Autodesk Inventor part; units mm, degrees
(part 3 of 3)
sketch "Эскиз6" plane through (0, 2, 0) normal (0, 1, 0) x (1, 0, 0)
  circle A0 centre (0, -40) radius 1.6 construction
  circle A1 centre (-46, 0) radius 1.6 construction
  circle A2 centre (46, 0) radius 1.6 construction
  line L0 (-6.25948, 46.133514) -> (-19.274559, 46.133514) construction
  arc A3 (-19.274559, 46.133514) -> (-21.669819, 47.125663) centre (-21.92031, 43.133514) ccw construction
  line L1 (-21.669819, 47.125663) -> (-42.426407, 67.882251) construction
  line L2 (-42.426407, 67.882251) -> (-34.294679, 76.013979) construction
  arc A4 (-34.294679, 76.013979) -> (-34.294679, 83.085047) centre (-37.830213, 79.549513) ccw construction
  line L3 (-34.294679, 83.085047) -> (-38.389169, 87.179537) construction
  arc A5 (-37.745267, 90.439454) -> (-38.389169, 87.179537) centre (-36.974956, 88.593751) ccw construction
  arc A6 (-25.810185, 94.54012) -> (-37.745267, 90.439454) centre (0, 0) ccw construction
  arc A7 (-25.810185, 94.54012) -> (-20.747604, 95.778583) centre (-24, 98.107084) ccw construction
  arc A8 (20.747604, 95.778583) -> (-20.747604, 95.778583) centre (0, 0) ccw construction
  arc A9 (20.747604, 95.778583) -> (25.810185, 94.54012) centre (24, 98.107084) ccw construction
  arc A10 (37.745267, 90.439454) -> (25.810185, 94.54012) centre (0, 0) ccw construction
  arc A11 (38.389169, 87.179537) -> (37.745267, 90.439454) centre (36.974956, 88.593751) ccw construction
  line L4 (38.389169, 87.179537) -> (34.294679, 83.085047) construction
  arc A12 (34.294679, 83.085047) -> (34.294679, 76.013979) centre (37.830213, 79.549513) ccw construction
  line L5 (34.294679, 76.013979) -> (42.426407, 67.882251) construction
  line L6 (42.426407, 67.882251) -> (21.669819, 47.125663) construction
  arc A13 (21.669819, 47.125663) -> (19.274559, 46.133514) centre (21.92031, 43.133514) ccw construction
  line L7 (19.274559, 46.133514) -> (6.25948, 46.133514) construction
  arc A14 (3.576846, 47.790579) -> (6.25948, 46.133514) centre (6.25948, 49.133514) ccw construction
  arc A15 (3.576846, 47.790579) -> (-3.576846, 47.790579) centre (0, 46) ccw construction
  arc A16 (-6.25948, 46.133514) -> (-3.576846, 47.790579) centre (-6.25948, 49.133514) ccw construction
  arc A17 (48.648149, 93.050296) -> (-48.648149, 93.050296) centre (0, 0) ccw construction
  arc A18 (-48.648149, 93.050296) -> (-49.379523, 88.270396) centre (-47.258202, 90.391716) ccw construction
  line L8 (-49.379523, 88.270396) -> (-46.315494, 85.206367) construction
  arc A19 (-46.315494, 73.892659) -> (-46.315494, 85.206367) centre (-51.972348, 79.549513) ccw construction
  line L9 (-46.315494, 73.892659) -> (-73.892659, 46.315494) construction
  arc A20 (-85.206367, 46.315494) -> (-73.892659, 46.315494) centre (-79.549513, 51.972348) ccw construction
  line L10 (-85.206367, 46.315494) -> (-88.270396, 49.379523) construction
  arc A21 (-88.270396, 49.379523) -> (-93.050296, 48.648149) centre (-90.391716, 47.258202) ccw
  arc A22 (-93.050296, 48.648149) -> (-93.050296, -48.648149) centre (0, 0) ccw construction
  arc A23 (-93.050296, -48.648149) -> (-88.270396, -49.379523) centre (-90.391716, -47.258202) ccw
  line L11 (-88.270396, -49.379523) -> (-85.206367, -46.315494) construction
  arc A24 (-73.892659, -46.315494) -> (-85.206367, -46.315494) centre (-79.549513, -51.972348) ccw construction
  line L12 (-73.892659, -46.315494) -> (-46.315494, -73.892659) construction
  arc A25 (-46.315494, -85.206367) -> (-46.315494, -73.892659) centre (-51.972348, -79.549513) ccw construction
  line L13 (-46.315494, -85.206367) -> (-49.379523, -88.270396) construction
  arc A26 (-49.379523, -88.270396) -> (-48.648149, -93.050296) centre (-47.258202, -90.391716) ccw construction
  arc A27 (-48.648149, -93.050296) -> (-45.41996, -94.667984) centre (0, 0) ccw construction
  arc A28 (-45.41996, -94.667984) -> (-43.035533, -94.165467) centre (-44.554817, -92.864785) ccw construction
  line L14 (-43.035533, -94.165467) -> (-18.380184, -65.366371) construction
  arc A29 (-17.477038, -64.764325) -> (-18.380184, -65.366371) centre (-16.8609, -66.667053) ccw construction
  line L15 (-17.477038, -64.764325) -> (-0.616138, -59.304458) construction
  arc A30 (0.616138, -59.304458) -> (-0.616138, -59.304458) centre (0, -61.207186) ccw construction
  line L16 (0.616138, -59.304458) -> (17.477038, -64.764325) construction
  arc A31 (18.380184, -65.366371) -> (17.477038, -64.764325) centre (16.8609, -66.667053) ccw construction
  line L17 (18.380184, -65.366371) -> (43.035533, -94.165467) construction
  arc A32 (43.035533, -94.165467) -> (45.41996, -94.667984) centre (44.554817, -92.864785) ccw construction
  arc A33 (45.41996, -94.667984) -> (48.648149, -93.050296) centre (0, 0) ccw construction
  arc A34 (48.648149, -93.050296) -> (49.379523, -88.270396) centre (47.258202, -90.391716) ccw construction
  line L18 (49.379523, -88.270396) -> (46.315494, -85.206367) construction
  arc A35 (46.315494, -73.892659) -> (46.315494, -85.206367) centre (51.972348, -79.549513) ccw construction
  line L19 (46.315494, -73.892659) -> (73.892659, -46.315494) construction
  arc A36 (85.206367, -46.315494) -> (73.892659, -46.315494) centre (79.549513, -51.972348) ccw construction
  line L20 (85.206367, -46.315494) -> (88.270396, -49.379523) construction
  arc A37 (88.270396, -49.379523) -> (93.050296, -48.648149) centre (90.391716, -47.258202) ccw construction
  arc A38 (93.050296, -48.648149) -> (93.050296, 48.648149) centre (0, 0) ccw construction
  arc A39 (93.050296, 48.648149) -> (88.270396, 49.379523) centre (90.391716, 47.258202) ccw construction
  line L21 (88.270396, 49.379523) -> (85.206367, 46.315494) construction
  arc A40 (73.892659, 46.315494) -> (85.206367, 46.315494) centre (79.549513, 51.972348) ccw construction
  line L22 (73.892659, 46.315494) -> (46.315494, 73.892659) construction
  arc A41 (46.315494, 85.206367) -> (46.315494, 73.892659) centre (51.972348, 79.549513) ccw construction
  line L23 (46.315494, 85.206367) -> (49.379523, 88.270396) construction
  arc A42 (49.379523, 88.270396) -> (48.648149, 93.050296) centre (47.258202, 90.391716) ccw construction
  circle A43 centre (-24, 98.107084) radius 1.6 construction
  arc A44 (47.790579, -3.576846) -> (46.133514, -6.25948) centre (49.133514, -6.25948) ccw construction
  arc A45 (47.790579, -3.576846) -> (47.790579, 3.576846) centre (46, 0) ccw construction
  arc A46 (46.133514, 6.25948) -> (47.790579, 3.576846) centre (49.133514, 6.25948) ccw construction
  line L24 (46.133514, 6.25948) -> (46.133514, 19.274559) construction
  arc A47 (46.133514, 19.274559) -> (47.125663, 21.669819) centre (43.133514, 21.92031) ccw construction
  line L25 (47.125663, 21.669819) -> (67.882251, 42.426407) construction
  line L26 (67.882251, 42.426407) -> (76.013979, 34.294679) construction
  arc A48 (76.013979, 34.294679) -> (83.085047, 34.294679) centre (79.549513, 37.830213) ccw construction
  line L27 (83.085047, 34.294679) -> (87.179537, 38.389169) construction
  arc A49 (90.439454, 37.745267) -> (87.179537, 38.389169) centre (88.593751, 36.974956) ccw construction
  arc A50 (97.965347, 2.605931) -> (90.439454, 37.745267) centre (0, 0) ccw construction
  arc A51 (97.965347, 2.605931) -> (97.965347, -2.605931) centre (101, 0) ccw construction
  arc A52 (90.439454, -37.745267) -> (97.965347, -2.605931) centre (0, 0) ccw construction
  arc A53 (87.179537, -38.389169) -> (90.439454, -37.745267) centre (88.593751, -36.974956) ccw construction
  line L28 (87.179537, -38.389169) -> (83.085047, -34.294679) construction
  arc A54 (83.085047, -34.294679) -> (76.013979, -34.294679) centre (79.549513, -37.830213) ccw construction
  line L29 (76.013979, -34.294679) -> (67.882251, -42.426407) construction
  line L30 (67.882251, -42.426407) -> (47.125663, -21.669819) construction
  arc A55 (47.125663, -21.669819) -> (46.133514, -19.274559) centre (43.133514, -21.92031) ccw construction
  line L31 (46.133514, -19.274559) -> (46.133514, -6.25948) construction
  circle A56 centre (101, 0) radius 1.6 construction
  circle A57 centre (-101, 0) radius 1.6 construction
  arc A58 (-47.790579, 3.576846) -> (-46.133514, 6.25948) centre (-49.133514, 6.25948) ccw construction
  arc A59 (-47.790579, 3.576846) -> (-47.790579, -3.576846) centre (-46, 0) ccw construction
  arc A60 (-46.133514, -6.25948) -> (-47.790579, -3.576846) centre (-49.133514, -6.25948) ccw construction
  line L32 (-46.133514, -6.25948) -> (-46.133514, -19.274559) construction
  arc A61 (-46.133514, -19.274559) -> (-47.125663, -21.669819) centre (-43.133514, -21.92031) ccw construction
  line L33 (-47.125663, -21.669819) -> (-67.882251, -42.426407) construction
  line L34 (-67.882251, -42.426407) -> (-76.013979, -34.294679) construction
  arc A62 (-76.013979, -34.294679) -> (-83.085047, -34.294679) centre (-79.549513, -37.830213) ccw construction
  line L35 (-83.085047, -34.294679) -> (-87.179537, -38.389169) construction
  arc A63 (-90.439454, -37.745267) -> (-87.179537, -38.389169) centre (-88.593751, -36.974956) ccw construction
  arc A64 (-97.965347, -2.605931) -> (-90.439454, -37.745267) centre (0, 0) ccw construction
  arc A65 (-97.965347, -2.605931) -> (-97.965347, 2.605931) centre (-101, 0) ccw construction
  arc A66 (-90.439454, 37.745267) -> (-97.965347, 2.605931) centre (0, 0) ccw construction
  arc A67 (-87.179537, 38.389169) -> (-90.439454, 37.745267) centre (-88.593751, 36.974956) ccw construction
  line L36 (-87.179537, 38.389169) -> (-83.085047, 34.294679) construction
  arc A68 (-83.085047, 34.294679) -> (-76.013979, 34.294679) centre (-79.549513, 37.830213) ccw construction
  line L37 (-76.013979, 34.294679) -> (-67.882251, 42.426407) construction
  line L38 (-67.882251, 42.426407) -> (-47.125663, 21.669819) construction
  arc A69 (-47.125663, 21.669819) -> (-46.133514, 19.274559) centre (-43.133514, 21.92031) ccw construction
  line L39 (-46.133514, 19.274559) -> (-46.133514, 6.25948) construction
  circle A70 centre (45.111051, -90.365885) radius 1.6 construction
  circle A71 centre (45.111051, 90.365885) radius 1.6 construction
  circle A72 centre (90.365885, 45.111051) radius 1.6 construction
  circle A73 centre (-45.111051, -90.365885) radius 1.6 construction
  circle A74 centre (90.365885, -45.111051) radius 1.6 construction
  circle A75 centre (-45.111051, 90.365885) radius 1.6 construction
  circle A76 centre (-90.365885, 45.111051) radius 1.6 construction
  circle A77 centre (-90.365885, -45.111051) radius 1.6 construction
  line L40 (63.63961, 46.669048) -> (43.84062, 26.870058) construction
  arc A78 (41.012193, 26.870058) -> (43.84062, 26.870058) centre (42.426407, 28.284271) ccw construction
  line L41 (41.012193, 26.870058) -> (26.870058, 41.012193) construction
  arc A79 (26.870058, 43.84062) -> (26.870058, 41.012193) centre (28.284271, 42.426407) ccw construction
  line L42 (26.870058, 43.84062) -> (46.669048, 63.63961) construction
  line L43 (46.669048, 63.63961) -> (63.63961, 46.669048) construction
  line L44 (-46.669048, 63.63961) -> (-26.870058, 43.84062) construction
  arc A80 (-26.870058, 41.012193) -> (-26.870058, 43.84062) centre (-28.284271, 42.426407) ccw construction
  line L45 (-26.870058, 41.012193) -> (-41.012193, 26.870058) construction
  arc A81 (-43.84062, 26.870058) -> (-41.012193, 26.870058) centre (-42.426407, 28.284271) ccw construction
  line L46 (-43.84062, 26.870058) -> (-63.63961, 46.669048) construction
  line L47 (-63.63961, 46.669048) -> (-46.669048, 63.63961) construction
  line L48 (-63.63961, -46.669048) -> (-43.84062, -26.870058) construction
  arc A82 (-41.012193, -26.870058) -> (-43.84062, -26.870058) centre (-42.426407, -28.284271) ccw construction
  line L49 (-41.012193, -26.870058) -> (-26.870058, -41.012193) construction
  arc A83 (-26.870058, -43.84062) -> (-26.870058, -41.012193) centre (-28.284271, -42.426407) ccw construction
  line L50 (-26.870058, -43.84062) -> (-46.669048, -63.63961) construction
  line L51 (-46.669048, -63.63961) -> (-63.63961, -46.669048) construction
  line L52 (-42.426407, -67.882251) -> (-21.669819, -47.125663) construction
  arc A84 (-21.669819, -47.125663) -> (-19.274559, -46.133514) centre (-21.92031, -43.133514) ccw construction
  line L53 (-19.274559, -46.133514) -> (19.274559, -46.133514) construction
  arc A85 (19.274559, -46.133514) -> (21.669819, -47.125663) centre (21.92031, -43.133514) ccw construction
  line L54 (21.669819, -47.125663) -> (42.426407, -67.882251) construction
  line L55 (42.426407, -67.882251) -> (37.124381, -73.184277) construction
  arc A86 (34.190883, -73.070746) -> (37.124381, -73.184277) centre (35.710168, -71.770063) ccw construction
  line L56 (34.190883, -73.070746) -> (25.418693, -62.824241) construction
  arc A87 (24.841986, -61.889251) -> (25.418693, -62.824241) centre (28.115423, -60.51553) ccw construction
  line L57 (24.841986, -61.889251) -> (23.83128, -59.480842) construction
  arc A88 (23.83128, -59.480842) -> (21.004883, -57.332824) centre (20.557843, -60.854564) ccw construction
  line L58 (21.004883, -57.332824) -> (15.158499, -56.590699) construction
  arc A89 (14.511894, -56.446301) -> (15.158499, -56.590699) centre (15.605539, -53.068959) ccw construction
  line L59 (14.511894, -56.446301) -> (0.616138, -51.946601) construction
  arc A90 (0.616138, -51.946601) -> (-0.616138, -51.946601) centre (0, -53.849329) ccw construction
  line L60 (-0.616138, -51.946601) -> (-14.511894, -56.446301) construction
  arc A91 (-15.158499, -56.590699) -> (-14.511894, -56.446301) centre (-15.605539, -53.068959) ccw construction
  line L61 (-15.158499, -56.590699) -> (-21.004883, -57.332824) construction
  arc A92 (-21.004883, -57.332824) -> (-23.83128, -59.480842) centre (-20.557843, -60.854564) ccw construction
  line L62 (-23.83128, -59.480842) -> (-24.841986, -61.889251) construction
  arc A93 (-25.418693, -62.824241) -> (-24.841986, -61.889251) centre (-28.115423, -60.51553) ccw construction
  line L63 (-25.418693, -62.824241) -> (-34.190883, -73.070746) construction
  arc A94 (-37.124381, -73.184277) -> (-34.190883, -73.070746) centre (-35.710168, -71.770063) ccw construction
  line L64 (-37.124381, -73.184277) -> (-42.426407, -67.882251) construction
  circle A95 centre (43.133514, 21.92031) radius 1.6 construction
  circle A96 centre (21.92031, -43.133514) radius 1.6 construction
  circle A97 centre (-21.92031, -43.133514) radius 1.6 construction
  circle A98 centre (-43.133514, -21.92031) radius 1.6 construction
  circle A99 centre (-43.133514, 21.92031) radius 1.6 construction
  circle A100 centre (-21.92031, 43.133514) radius 1.6 construction
  circle A101 centre (43.133514, -21.92031) radius 1.6 construction
  circle A102 centre (21.92031, 43.133514) radius 1.6 construction
  circle A103 centre (-37.830213, 79.549513) radius 1.6 construction
  circle A104 centre (-79.549513, 37.830213) radius 1.6 construction
  circle A105 centre (-79.549513, -37.830213) radius 1.6 construction
  circle A106 centre (79.549513, -37.830213) radius 1.6 construction
  circle A107 centre (37.830213, 79.549513) radius 1.6 construction
  circle A108 centre (79.549513, 37.830213) radius 1.6 construction
  circle A109 centre (-20.557843, -60.854564) radius 1.55 construction
  circle A110 centre (20.557843, -60.854564) radius 1.55 construction
  circle A111 centre (37.830213, -79.549513) radius 1.6 construction
  circle A112 centre (-37.830213, -79.549513) radius 1.6 construction
  line L65 (46.669048, -63.63961) -> (26.870058, -43.84062) construction
  arc A113 (26.870058, -41.012193) -> (26.870058, -43.84062) centre (28.284271, -42.426407) ccw construction
  line L66 (26.870058, -41.012193) -> (41.012193, -26.870058) construction
  arc A114 (43.84062, -26.870058) -> (41.012193, -26.870058) centre (42.426407, -28.284271) ccw construction
  line L67 (43.84062, -26.870058) -> (63.63961, -46.669048) construction
  line L68 (63.63961, -46.669048) -> (46.669048, -63.63961) construction
  circle A115 centre (24, 98.107084) radius 1.6 construction
  circle A116 centre (0, 46) radius 1.6 construction
  arc A117 (3.649244, -38.362008) -> (6.386177, -40.133514) centre (6.386177, -37.133514) ccw construction
  arc A118 (3.649244, -38.362008) -> (-3.649244, -38.362008) centre (0, -40) ccw construction
  arc A119 (-6.386177, -40.133514) -> (-3.649244, -38.362008) centre (-6.386177, -37.133514) ccw construction
  line L69 (-6.386177, -40.133514) -> (-19.274559, -40.133514) construction
  arc A120 (-19.274559, -40.133514) -> (-21.669819, -39.141365) centre (-21.92031, -43.133514) ccw construction
  line L70 (-21.669819, -39.141365) -> (-39.141365, -21.669819) construction
  arc A121 (-39.141365, -21.669819) -> (-40.133514, -19.274559) centre (-43.133514, -21.92031) ccw construction
  line L71 (-40.133514, -19.274559) -> (-40.133514, 19.274559) construction
  arc A122 (-40.133514, 19.274559) -> (-39.141365, 21.669819) centre (-43.133514, 21.92031) ccw construction
  line L72 (-39.141365, 21.669819) -> (-21.669819, 39.141365) construction
  arc A123 (-21.669819, 39.141365) -> (-19.274559, 40.133514) centre (-21.92031, 43.133514) ccw construction
  line L73 (-19.274559, 40.133514) -> (19.274559, 40.133514) construction
  arc A124 (19.274559, 40.133514) -> (21.669819, 39.141365) centre (21.92031, 43.133514) ccw construction
  line L74 (21.669819, 39.141365) -> (39.141365, 21.669819) construction
  arc A125 (39.141365, 21.669819) -> (40.133514, 19.274559) centre (43.133514, 21.92031) ccw construction
  line L75 (40.133514, 19.274559) -> (40.133514, -19.274559) construction
  arc A126 (40.133514, -19.274559) -> (39.141365, -21.669819) centre (43.133514, -21.92031) ccw construction
  line L76 (39.141365, -21.669819) -> (21.669819, -39.141365) construction
  arc A127 (21.669819, -39.141365) -> (19.274559, -40.133514) centre (21.92031, -43.133514) ccw construction
  line L77 (19.274559, -40.133514) -> (6.386177, -40.133514) construction
  arc A128 (-93.669434, -39.093312) -> (-84.704663, -40.864043) centre (-88.593751, -36.974956) ccw construction
  line L78 (-84.704663, -40.864043) -> (-80.610173, -36.769553) construction
  arc A129 (-78.488853, -36.769553) -> (-80.610173, -36.769553) centre (-79.549513, -37.830213) ccw construction
  line L79 (-78.488853, -36.769553) -> (-67.882251, -47.376154) construction
  line L80 (-67.882251, -47.376154) -> (-42.77996, -22.273864) construction
  arc A130 (-42.633514, -21.92031) -> (-42.77996, -22.273864) centre (-43.133514, -21.92031) ccw construction
  line L81 (-42.633514, -21.92031) -> (-42.633514, -6.25948) construction
  line L82 (-42.633514, 6.25948) -> (-42.633514, 21.92031) construction
  arc A131 (-42.77996, 22.273864) -> (-42.633514, 21.92031) centre (-43.133514, 21.92031) ccw construction
  line L83 (-42.77996, 22.273864) -> (-67.882251, 47.376154) construction
  line L84 (-67.882251, 47.376154) -> (-78.488853, 36.769553) construction
  arc A132 (-80.610173, 36.769553) -> (-78.488853, 36.769553) centre (-79.549513, 37.830213) ccw construction
  line L85 (-80.610173, 36.769553) -> (-84.704663, 40.864043) construction
  arc A133 (-101, -3.5) -> (-101.369276, 3.480465) centre (-101, 0) ccw
  arc A134 (-93.050296, 48.648149) -> (-93.050296, -48.648149) centre (0, 0) ccw construction
  arc A135 (-105, 0) -> (-93.050296, -48.648149) centre (0, 0) ccw
  arc A136 (-93.050296, 48.648149) -> (-105, 0) centre (0, 0) ccw
  line L86 (-88.270396, -49.379523) -> (-85.206367, -46.315494)
  line L87 (-90.439454, -37.745267) -> (-90.419699, -37.79099)
  circle A137 centre (-101, 0) radius 1.5
  circle A138 centre (-90.365885, 45.111051) radius 1.5
  circle A139 centre (-90.365885, -45.111051) radius 1.5
  line L88 (-160.503485, 209.293853) -> (164.91253, 209.293853)
  line L89 (164.91253, 209.293853) -> (164.91253, -147.440984)
  line L90 (164.91253, -147.440984) -> (-160.503485, -147.440984)
  line L91 (-160.503485, -147.440984) -> (-160.503485, 209.293853)
  arc A140 (-89.82793, 38.548741) -> (-88.458528, -41.595089) centre (0, 0) ccw construction
  arc A141 (-93.664396, 42.848348) -> (-88.458528, 41.595089) centre (-90.365885, 45.111051) ccw
  arc A142 (-88.270396, 49.379523) -> (-93.050296, 48.648149) centre (-90.391716, 47.258202) ccw
  line L92 (-88.270396, 49.379523) -> (-85.773457, 46.882584)
  circle A143 centre (-46, 0) radius 1.6 construction
  line L93 (-46, 0) -> (46, 0) construction
  arc A144 (-88.458528, -41.595089) -> (-93.664396, -42.848348) centre (-90.365885, -45.111051) ccw
  arc A145 (-88.458528, 41.595089) -> (-89.82793, 38.548741) centre (0, 0) ccw construction
  arc A146 (-85.773457, 46.882584) -> (-88.458528, 41.595089) centre (0, 0) ccw
  arc A147 (-88.458528, -41.595089) -> (-85.773457, -46.882584) centre (0, 0) ccw
  arc A148 (-85.773457, -46.882584) -> (-85.773457, 46.882584) centre (0, 0) ccw construction
  arc A149 (-102.940517, -3.5) -> (-93.664396, -42.848348) centre (0, 0) ccw
  line L94 (-101, -3.5) -> (-102.940517, -3.5)
  line L95 (-46, 0) -> (-101, 0) construction
  line L96 (-101, 3.5) -> (-102.940517, 3.5)
  arc A150 (-102.940517, 3.5) -> (-102.940517, -3.5) centre (0, 0) ccw construction
  arc A151 (-93.664396, 42.848348) -> (-102.940517, 3.5) centre (0, 0) ccw
  arc A152 (-93.664396, -42.848348) -> (-93.664396, 42.848348) centre (0, 0) ccw construction
  point P0 (-101, 3.5)
  dimension "d112" = 7
  dimension "d115" = 105
  dimension "d116" = 105
  dimension "d119" = 3
  dimension "d120" = 3
  dimension "d121" = 3
  dimension "d126" = 195.5
  dimension "d128" = 4
  dimension "d139" = 2
  constraints: 44 point on circle, 36 end point, 22 centre point, 6 coincident, 4 symmetric about line, 3 horizontal, 3 parallel, 2 point on line, 1 perpendicular, 1 tangent, 12 other
  measures "d112" diameter of A133
  measures "d115" radius of A135
  measures "d116" radius of A136
  measures "d119" diameter of A137
  measures "d120" diameter of A138
  measures "d121" diameter of A139
  measures "d126" diameter of A140
  measures "d128" radius of A141
  measures "d139" radial gap between concentric circles of A22 A149
extrude "Выдавливание9" add sketch "Эскиз6" along normal blind 35 contours L92 A146 A141 A151 L96 A133 L94 A149 A144 A147 L86 A23 A135 A136 A21
extrude "Выдавливание10" cut sketch "Эскиз6" against normal blind 10 contours L92 A146 A141 A151 L96 A133 L94 A149 A144 A147 L86 A23 A135 A136 A21 | A137 | A138 | A139 | L88 L89 L90 L91
fillet "Сопряжение1" radius 2 4 edges at (-85.7735, 19.5, -46.8826) (-85.7735, 19.5, 46.8826) (-88.4585, 19.5, 41.5951) (-88.4585, 19.5, -41.5951)
ref_plane "РабПлоскость2" through (-105, 2, 0) normal (1, 0, 0) x (0, 1, 0)
ref_plane "РабПлоскость3" through (-86.469284, 2, -45.586461) normal (-1, 0, 0) x (0, -1, 0)
sketch "Эскиз10" plane through (0, 0, 0) normal (0, 0, 1) x (1, 0, 0)
  line L0 (-97.5, 2) -> (-97.5, 37) construction
  line L1 (-96.322071, 38.959767) -> (-77.348594, 6.096741) construction
  point P0 (0, 0)
  dimension "d157" = 30
  dimension "d158" = 2
  constraints: 2 end point
  measures "d157" angle of L0 L1
  measures "d158" distance from line of L0.end L1
sketch "Эскиз11" plane through (-86.469284, 2, -45.586461) normal (-1, 0, 0) x (0, -1, 0)
  line L0 (-33.2, 80.586461) -> (-2, 80.586461)
  line L1 (-2, 80.586461) -> (-2, 10.586461)
  line L2 (-2, 10.586461) -> (-33.2, 10.586461)
  line L3 (-33.2, 10.586461) -> (-33.2, 80.586461)
  line L4 (-33.2, 45.586461) -> (-2, 45.586461) construction
  line L5 (-17.6, 10.586461) -> (-17.6, 80.586461) construction
  line L6 (-35, 44.086461) -> (-35, 47.086461) construction
  line L7 (0, 44.086461) -> (0, 47.086461) construction
  line L8 (0, 45.586461) -> (-35, 45.586461) construction
  point P0 (2, 45.586461)
  dimension "d154" = 70
  dimension "d155" = 31.2
  dimension "d156" = 2
  constraints: 14 end point, 6 midpoint, 2 parallel, 1 collinear, 1 horizontal, 1 perpendicular
  measures "d154" distance of L2.end L0.start
  measures "d155" distance of L1.end L2.end
  measures "d156" distance between parallel lines of L7 L1
ref_plane "РабПлоскость4" through (-96.322071, 38.959767, 0) normal (0.8660254, 0.5, 0) x (0.5, -0.8660254, 0)
ref_plane "РабПлоскость5" through (0, 2, 0) normal (0, -1, 0) x (1, 0, 0)
ref_plane "РабПлоскость6" through (0, 37, 0) normal (0, 1, 0) x (1, 0, 0)
sketch "Эскиз12" plane through (-96.322071, 38.959767, 0) normal (0.8660254, 0.5, 0) x (0.5, -0.8660254, 0)
  line L0 (4.677462, -35) -> (40.677462, -35) construction
  line L1 (40.677462, -35) -> (40.677462, 35.3) construction
  line L2 (40.677462, 35.3) -> (4.677462, 35.3) construction
  line L3 (4.677462, 35.3) -> (4.677462, -35) construction
  ellipse E0 centre (-0.641757, 0) end of major axis (-0.641757, 1.5) minor radius 0.75 construction
  ellipse E1 centre (4.675301, -45.111051) end of major axis (4.675301, -43.611051) minor radius 0.75 construction
  ellipse E2 centre (4.675301, 45.111051) end of major axis (4.675301, 46.611051) minor radius 0.75 construction
  ellipse E3 centre (4.893407, 43.159201) end of major axis (4.893407, 41.159201) minor radius 1 (5.111513, 41.207351) -> (5.794958, 42.293853) ccw construction
  ellipse E4 centre (49.858243, 0) end of major axis (49.858243, -97.75) minor radius 48.875 (6.623601, 45.586461) -> (5.794958, 42.293853) ccw construction
  ellipse E5 centre (5.739005, 46.519176) end of major axis (5.739005, 44.519176) minor radius 1 (6.623601, 45.586461) -> (6.446111, 47.93339) ccw construction
  line L4 (6.446111, 47.93339) -> (5.723045, 49.379523) construction
  ellipse E6 centre (4.662385, 47.258202) end of major axis (4.662385, 50.258202) minor radius 1.5 (5.723045, 49.379523) -> (3.333095, 48.648149) ccw construction
  ellipse E7 centre (49.858243, 0) end of major axis (49.858243, -105) minor radius 52.5 (3.333095, 48.648149) -> (3.333095, -48.648149) ccw construction
  ellipse E8 centre (4.662385, -47.258202) end of major axis (4.662385, -50.258202) minor radius 1.5 (3.333095, -48.648149) -> (5.723045, -49.379523) ccw construction
  line L5 (5.723045, -49.379523) -> (6.446111, -47.93339) construction
  ellipse E9 centre (5.739005, -46.519176) end of major axis (5.739005, -48.519176) minor radius 1 (6.446111, -47.93339) -> (6.623601, -45.586461) ccw construction
  ellipse E10 centre (49.858243, 0) end of major axis (49.858243, -97.75) minor radius 48.875 (5.794958, -42.293853) -> (6.623601, -45.586461) ccw construction
  ellipse E11 centre (4.893407, -43.159201) end of major axis (4.893407, -45.159201) minor radius 1 (5.794958, -42.293853) -> (5.111513, -41.207351) ccw construction
  ellipse E12 centre (4.675301, -45.111051) end of major axis (4.675301, -41.111051) minor radius 2 (5.111513, -41.207351) -> (3.026045, -42.848348) ccw construction
  ellipse E13 centre (49.858243, 0) end of major axis (49.858243, -103) minor radius 51.5 (-1.612015, -3.5) -> (3.026045, -42.848348) ccw construction
  line L6 (-1.612015, -3.5) -> (-0.641757, -3.5) construction
  ellipse E14 centre (-0.641757, 0) end of major axis (-0.641757, -3.5) minor radius 1.75 (-0.641757, -3.5) -> (-0.641757, 3.5) ccw construction
  line L7 (-0.641757, 3.5) -> (-1.612015, 3.5) construction
  ellipse E15 centre (49.858243, 0) end of major axis (49.858243, -103) minor radius 51.5 (3.026045, 42.848348) -> (-1.612015, 3.5) ccw construction
  ellipse E16 centre (4.675301, 45.111051) end of major axis (4.675301, 41.111051) minor radius 2 (3.026045, 42.848348) -> (5.111513, 41.207351) ccw construction
  ellipse E17 centre (49.858243, 0) end of major axis (49.858243, -105) minor radius 52.5 (3.333095, 48.648149) -> (3.333095, -48.648149) ccw construction
  ellipse E18 centre (49.858243, 0) end of major axis (49.858243, -103) minor radius 51.5 (-1.612015, -3.5) -> (3.026045, -42.848348) ccw construction
  ellipse E19 centre (49.858243, 0) end of major axis (49.858243, -103) minor radius 51.5 (3.026045, 42.848348) -> (-1.612015, 3.5) ccw construction
  line L8 (2.262943, 70.716347) -> (2.262943, -70.716347) construction
  line L9 (42.677462, 70.716347) -> (42.677462, -70.716347) construction
  line L10 (4.677462, 0.15) -> (40.677462, 0.15) construction
  line L11 (0, 0) -> (37.946953, 0) construction
  circle A0 centre (7.177462, -31) radius 1.9
  line L12 (22.677462, -35) -> (22.677462, 35.3) construction
  circle A1 centre (38.177462, -31) radius 1.9
  circle A2 centre (7.302462, 31.05) radius 1.9
  circle A3 centre (38.052462, 31.05) radius 1.9
  line L13 (5.177462, -35) -> (9.177462, -35)
  line L14 (11.177462, -33) -> (11.177462, -29)
  line L15 (9.177462, -27) -> (5.177462, -27)
  line L16 (3.177462, -29) -> (3.177462, -33)
  arc A4 (9.177462, -35) -> (11.177462, -33) centre (9.177462, -33) ccw
  arc A5 (3.177462, -33) -> (5.177462, -35) centre (5.177462, -33) ccw
  arc A6 (5.177462, -27) -> (3.177462, -29) centre (5.177462, -29) ccw
  arc A7 (11.177462, -29) -> (9.177462, -27) centre (9.177462, -29) ccw
  line L17 (40.177462, -35) -> (36.177462, -35)
  line L18 (34.177462, -33) -> (34.177462, -29)
  line L19 (36.177462, -27) -> (40.177462, -27)
  arc A8 (34.177462, -33) -> (36.177462, -35) centre (36.177462, -33) ccw
  arc A9 (40.177462, -35) -> (42.177462, -33) centre (40.177462, -33) ccw
  arc A10 (42.177462, -29) -> (40.177462, -27) centre (40.177462, -29) ccw
  arc A11 (36.177462, -27) -> (34.177462, -29) centre (36.177462, -29) ccw
  line L20 (42.177462, -29) -> (42.177462, -33)
  line L21 (5.302462, 27.05) -> (9.302462, 27.05)
  line L22 (11.302462, 29.05) -> (11.302462, 33.05)
  line L23 (9.302462, 35.05) -> (5.302462, 35.05)
  line L24 (3.302462, 33.05) -> (3.302462, 29.05)
  arc A12 (9.302462, 27.05) -> (11.302462, 29.05) centre (9.302462, 29.05) ccw
  arc A13 (11.302462, 33.05) -> (9.302462, 35.05) centre (9.302462, 33.05) ccw
  arc A14 (5.302462, 35.05) -> (3.302462, 33.05) centre (5.302462, 33.05) ccw
  arc A15 (3.302462, 29.05) -> (5.302462, 27.05) centre (5.302462, 29.05) ccw
  line L25 (40.052462, 27.05) -> (36.052462, 27.05)
  line L26 (34.052462, 29.05) -> (34.052462, 33.05)
  line L27 (36.052462, 35.05) -> (40.052462, 35.05)
  line L28 (42.052462, 33.05) -> (42.052462, 29.05)
  arc A16 (34.052462, 29.05) -> (36.052462, 27.05) centre (36.052462, 29.05) ccw
  arc A17 (36.052462, 35.05) -> (34.052462, 33.05) centre (36.052462, 33.05) ccw
  arc A18 (42.052462, 33.05) -> (40.052462, 35.05) centre (40.052462, 33.05) ccw
  arc A19 (40.052462, 27.05) -> (42.052462, 29.05) centre (40.052462, 29.05) ccw
  point P0 (81.901183, 0)
  point P1 (2.271019, -44.348896)
  point P2 (2.271019, -39.38051)
  point P3 (2.274211, 39.395934)
  point P4 (7.177462, -32.9)
  point P5 (7.302462, 32.95)
  point P6 (11.302462, 35.05)
  point P7 (11.302462, 27.05)
  point P8 (3.302462, 35.05)
  dimension "d166" = 3.8
  dimension "d169" = 3.8
  dimension "d160" = 36
  dimension "d161" = 70.3
  dimension "d164" = 2
  dimension "d165" = 0.15
  dimension "d167" = 31
  dimension "d168" = 4
  dimension "d170" = 30.75
  dimension "d171" = 4.25
  dimension "d172" = 4
  dimension "d173" = 4
  dimension "d174" = 4
  dimension "d175" = 4
  dimension "d176" = 2
  dimension "d177" = 8
  dimension "d178" = 8
  dimension "d179" = 4
  dimension "d180" = 4
  dimension "d181" = 2
  dimension "d182" = 2
  constraints: 44 end point, 32 point on circle, 26 symmetric about line, 18 centre point, 16 tangent, 6 parallel, 6 point on line, 5 equal radius, 4 midpoint, 3 horizontal, 3 perpendicular, 2 vertical alignment, 36 other
  measures "d160" distance of L1.end L2.end
  measures "d161" distance of L2.end L0.start
  measures "d164" distance between parallel lines of L9 L1
  measures "d165" distance between parallel lines of L11 L10
  measures "d167" distance of A1.centre point (7.177, -31)
  measures "d168" distance from line of L0 point (7.177, -31)
  measures "d170" distance of A3.centre point (7.302, 31.05)
  measures "d171" distance from line of L2 point (7.302, 31.05)
  measures "d172" distance from line of point (7.177, -31) L15
  measures "d173" distance from line of point (7.177, -31) L13
  measures "d174" distance from line of point (7.177, -31) L16
  measures "d175" distance from line of point (7.177, -31) L14
  measures "d176" radius of A4
  measures "d177" distance of point (3.302, 35.05) point (11.302, 35.05)
  measures "d178" distance of point (11.302, 35.05) point (11.302, 27.05)
  measures "d179" distance from line of L24 point (7.302, 31.05)
  measures "d180" distance from line of L21 point (7.302, 31.05)
  measures "d181" radius of A12
  measures "d182" radius of A15
extrude "Выдавливание12" add sketch "Эскиз12" against normal blind 4
sketch "Эскиз8" plane through (-105, 2, 0) normal (1, 0, 0) x (0, 1, 0)
  line L0 (0, -48.648149) -> (0, 48.648149) construction
  line L1 (0, 48.648149) -> (35, 48.648149) construction
  line L2 (35, -48.648149) -> (35, 48.648149) construction
  line L3 (0, -48.648149) -> (35, -48.648149) construction
  line L4 (0, 48.648149) -> (0, 49.379523) construction
  line L5 (0, 49.379523) -> (35, 49.379523) construction
  line L6 (35, 48.648149) -> (35, 49.379523) construction
  line L7 (0, 48.648149) -> (35, 48.648149) construction
  line L8 (0, -49.379523) -> (0, -48.648149) construction
  line L9 (0, -48.648149) -> (35, -48.648149) construction
  line L10 (35, -49.379523) -> (35, -48.648149) construction
  line L11 (0, -49.379523) -> (35, -49.379523) construction
  line L12 (0, -48.648149) -> (35, -48.648149) construction
  line L13 (0, 48.648149) -> (35, 48.648149) construction
  line L14 (35, -48.648149) -> (0, 48.648149) construction
  line L15 (35, 48.648149) -> (0, -48.648149) construction
  line L16 (11.700962, 7.044229) -> (20.700962, -8.544229)
  line L17 (20.700962, -8.544229) -> (23.299038, -7.044229)
  line L18 (23.299038, -7.044229) -> (14.299038, 8.544229)
  line L19 (14.299038, 8.544229) -> (11.700962, 7.044229)
  line L20 (11.700962, 7.044229) -> (23.299038, -7.044229) construction
  line L21 (20.700962, -8.544229) -> (14.299038, 8.544229) construction
  line L22 (35, -48.648149) -> (35, 48.648149) construction
  line L23 (35, 0) -> (0, 0) construction
  line L24 (11.700962, -7.044229) -> (14.299038, -8.544229)
  line L25 (23.299038, 7.044229) -> (20.700962, 8.544229)
  line L26 (20.700962, 8.544229) -> (11.700962, -7.044229)
  line L27 (14.299038, -8.544229) -> (20.700962, 8.544229) construction
  line L28 (23.299038, 7.044229) -> (11.700962, -7.044229) construction
  line L29 (14.299038, -8.544229) -> (23.299038, 7.044229)
  line L30 (26.5, -1.5) -> (26.5, 1.5)
  line L31 (8.5, 1.5) -> (8.5, -1.5)
  line L32 (8.5, -1.5) -> (26.5, -1.5)
  line L33 (26.5, 1.5) -> (8.5, -1.5) construction
  line L34 (8.5, 1.5) -> (26.5, -1.5) construction
  line L35 (26.5, 1.5) -> (8.5, 1.5)
  point P0 (-2, 0)
  point P1 (17.5, 0)
  point P2 (17.5, 0)
  point P3 (17.5, 0)
  point P4 (14.901924, 1.5)
  point P5 (14.901924, -1.5)
  point P6 (17.5, -3)
  point P7 (20.098076, -1.5)
  point P8 (20.098076, 1.5)
  point P9 (17.5, 3)
  dimension "d143" = 3
  dimension "d144" = 18
  dimension "d145" = 60
  dimension "d148" = 360
  constraints: 42 end point, 9 midpoint, 2 coincident, 2 parallel, 1 perpendicular, 32 other
  measures "d143" distance of L17.end L16.end
  measures "d144" distance of L17.end L18.end
  measures "d145" angle of L23 L18
extrude "asterisk" cut sketch "Эскиз8" along normal blind 0.6
ref_plane "РабПлоскость7" through (-94.73334, 36.208003, 31) normal (1, 0, 0) x (0, 1, 0)
sketch "Эскиз13" plane through (-94.73334, 36.208003, 31) normal (1, 0, 0) x (0, 1, 0)
  ellipse E0 centre (-1.732051, -2) end of major axis (-1.732051, -4) minor radius 1.732051 (-1.732051, -4) -> (0, -2) ccw
  line L0 (0, -2) -> (0, 2)
  ellipse E1 centre (-1.732051, 2) end of major axis (-1.732051, 4) minor radius 1.732051 (0, 2) -> (-1.732051, 4) ccw
  line L1 (-1.732051, 4) -> (-5.196152, 4)
  ellipse E2 centre (-5.196152, 2) end of major axis (-5.196152, 4) minor radius 1.732051 (-5.196152, 4) -> (-6.928203, 2) ccw construction
  line L2 (-6.928203, 2) -> (-6.928203, -2) construction
  ellipse E3 centre (-5.196152, -2) end of major axis (-5.196152, -4) minor radius 1.732051 (-6.928203, -2) -> (-5.196152, -4) ccw construction
  line L3 (-5.196152, -4) -> (-1.732051, -4)
  ellipse E4 centre (-3.464102, 0) end of major axis (-3.464102, -1.9) minor radius 1.645448 construction
  ellipse E5 centre (-28.578838, -2) end of major axis (-28.578838, -4) minor radius 1.732051 (-28.578838, -4) -> (-26.846788, -2) ccw construction
  line L4 (-26.846788, -2) -> (-26.846788, 2) construction
  ellipse E6 centre (-28.578838, 2) end of major axis (-28.578838, 4) minor radius 1.732051 (-26.846788, 2) -> (-28.578838, 4) ccw construction
  line L5 (-28.578838, 4) -> (-32.04294, 4)
  ellipse E7 centre (-32.04294, 2) end of major axis (-32.04294, 4) minor radius 1.732051 (-32.04294, 4) -> (-33.774991, 2) ccw
  line L6 (-33.774991, 2) -> (-33.774991, -2)
  ellipse E8 centre (-32.04294, -2) end of major axis (-32.04294, -4) minor radius 1.732051 (-33.774991, -2) -> (-32.04294, -4) ccw
  line L7 (-32.04294, -4) -> (-28.578838, -4)
  ellipse E9 centre (-30.310889, 0) end of major axis (-30.310889, -1.9) minor radius 1.645448 construction
  line L8 (-33.774991, 2) -> (-33.774991, -2) construction
  line L9 (-33.774991, 2) -> (-35.774991, 2) construction
  line L10 (-35.774991, -2) -> (-35.774991, 2)
  line L11 (-33.774991, -2) -> (-35.774991, -2) construction
  ellipse E10 centre (-32.04294, -2) end of major axis (-32.04294, -4) minor radius 1.732051 (-33.774991, -2) -> (-32.04294, -4) ccw construction
  line L12 (-33.774991, -2) -> (-35.774991, -2) construction
  ellipse E11 centre (-34.04294, -2) end of major axis (-34.04294, 0) minor radius 1.732051 (-35.774991, -2) -> (-34.04294, -4) ccw
  line L13 (-32.04294, -4) -> (-34.04294, -4) construction
  ellipse E12 centre (-32.04294, 2) end of major axis (-32.04294, 4) minor radius 1.732051 (-32.04294, 4) -> (-33.774991, 2) ccw construction
  line L14 (-32.04294, 4) -> (-34.04294, 4) construction
  ellipse E13 centre (-34.04294, 2) end of major axis (-34.04294, 4) minor radius 1.732051 (-34.04294, 4) -> (-35.774991, 2) ccw
  line L15 (-33.774991, 2) -> (-35.774991, 2) construction
  ellipse E14 centre (-5.196152, 2) end of major axis (-5.196152, 4) minor radius 1.732051 (-5.196152, 4) -> (-6.928203, 2) ccw construction
  line L16 (-5.196152, 4) -> (-7.196152, 4) construction
  ellipse E15 centre (-7.196152, 2) end of major axis (-7.196152, 4) minor radius 1.732051 (-7.196152, 4) -> (-8.928203, 2) ccw
  line L17 (-6.928203, 2) -> (-8.928203, 2) construction
  line L18 (-6.928203, 2) -> (-6.928203, -2) construction
  line L19 (-6.928203, 2) -> (-8.928203, 2) construction
  line L20 (-8.928203, -2) -> (-8.928203, 2)
  line L21 (-6.928203, -2) -> (-8.928203, -2) construction
  ellipse E16 centre (-5.196152, -2) end of major axis (-5.196152, -4) minor radius 1.732051 (-6.928203, -2) -> (-5.196152, -4) ccw construction
  line L22 (-6.928203, -2) -> (-8.928203, -2) construction
  ellipse E17 centre (-7.196152, -2) end of major axis (-7.196152, 0) minor radius 1.732051 (-8.928203, -2) -> (-7.196152, -4) ccw
  line L23 (-5.196152, -4) -> (-7.196152, -4)
  ellipse E18 centre (-5.304406, -64.05) end of major axis (-5.304406, -66.05) minor radius 1.732051 (-7.036456, -64.05) -> (-5.304406, -66.05) ccw construction
  line L24 (-5.304406, -66.05) -> (-1.840304, -66.05)
  ellipse E19 centre (-1.840304, -64.05) end of major axis (-1.840304, -66.05) minor radius 1.732051 (-1.840304, -66.05) -> (-0.108253, -64.05) ccw
  line L25 (-0.108253, -64.05) -> (-0.108253, -60.05)
  ellipse E20 centre (-1.840304, -60.05) end of major axis (-1.840304, -58.05) minor radius 1.732051 (-0.108253, -60.05) -> (-1.840304, -58.05) ccw
  line L26 (-1.840304, -58.05) -> (-5.304406, -58.05)
  ellipse E21 centre (-5.304406, -60.05) end of major axis (-5.304406, -58.05) minor radius 1.732051 (-5.304406, -58.05) -> (-7.036456, -60.05) ccw construction
  line L27 (-7.036456, -60.05) -> (-7.036456, -64.05) construction
  ellipse E22 centre (-3.572355, -62.05) end of major axis (-3.572355, -63.95) minor radius 1.645448 construction
  line L28 (-7.036456, -60.05) -> (-7.036456, -64.05) construction
  line L29 (-7.036456, -60.05) -> (-9.036456, -60.05) construction
  line L30 (-9.036456, -64.05) -> (-9.036456, -60.05)
  line L31 (-7.036456, -64.05) -> (-9.036456, -64.05) construction
  ellipse E23 centre (-5.304406, -60.05) end of major axis (-5.304406, -58.05) minor radius 1.732051 (-5.304406, -58.05) -> (-7.036456, -60.05) ccw construction
  line L32 (-5.304406, -58.05) -> (-7.304406, -58.05) construction
  ellipse E24 centre (-7.304406, -60.05) end of major axis (-7.304406, -58.05) minor radius 1.732051 (-7.304406, -58.05) -> (-9.036456, -60.05) ccw
  line L33 (-7.036456, -60.05) -> (-9.036456, -60.05) construction
  ellipse E25 centre (-5.304406, -64.05) end of major axis (-5.304406, -66.05) minor radius 1.732051 (-7.036456, -64.05) -> (-5.304406, -66.05) ccw construction
  line L34 (-7.036456, -64.05) -> (-9.036456, -64.05) construction
  ellipse E26 centre (-7.304406, -64.05) end of major axis (-7.304406, -62.05) minor radius 1.732051 (-9.036456, -64.05) -> (-7.304406, -66.05) ccw
  line L35 (-5.304406, -66.05) -> (-7.304406, -66.05) construction
  ellipse E27 centre (-28.470585, -60.05) end of major axis (-28.470585, -58.05) minor radius 1.732051 (-26.738534, -60.05) -> (-28.470585, -58.05) ccw construction
  line L36 (-28.470585, -58.05) -> (-31.934687, -58.05)
  ellipse E28 centre (-31.934687, -60.05) end of major axis (-31.934687, -58.05) minor radius 1.732051 (-31.934687, -58.05) -> (-33.666738, -60.05) ccw
  line L37 (-33.666738, -60.05) -> (-33.666738, -64.05)
  ellipse E29 centre (-31.934687, -64.05) end of major axis (-31.934687, -66.05) minor radius 1.732051 (-33.666738, -64.05) -> (-31.934687, -66.05) ccw
  line L38 (-31.934687, -66.05) -> (-28.470585, -66.05)
  ellipse E30 centre (-28.470585, -64.05) end of major axis (-28.470585, -66.05) minor radius 1.732051 (-28.470585, -66.05) -> (-26.738534, -64.05) ccw construction
  line L39 (-26.738534, -64.05) -> (-26.738534, -60.05) construction
  ellipse E31 centre (-30.202636, -62.05) end of major axis (-30.202636, -63.95) minor radius 1.645448 construction
  ellipse E32 centre (-31.934687, -64.05) end of major axis (-31.934687, -66.05) minor radius 1.732051 (-33.666738, -64.05) -> (-31.934687, -66.05) ccw construction
  line L40 (-33.666738, -64.05) -> (-35.666738, -64.05) construction
  ellipse E33 centre (-33.934687, -64.05) end of major axis (-33.934687, -62.05) minor radius 1.732051 (-35.666738, -64.05) -> (-33.934687, -66.05) ccw
  line L41 (-31.934687, -66.05) -> (-33.934687, -66.05) construction
  line L42 (-33.666738, -60.05) -> (-33.666738, -64.05) construction
  line L43 (-33.666738, -60.05) -> (-33.666738, -64.05) construction
  line L44 (-33.666738, -60.05) -> (-35.666738, -60.05) construction
  line L45 (-35.666738, -64.05) -> (-35.666738, -60.05) construction
  line L46 (-33.666738, -64.05) -> (-35.666738, -64.05) construction
  ellipse E34 centre (-31.934687, -60.05) end of major axis (-31.934687, -58.05) minor radius 1.732051 (-31.934687, -58.05) -> (-33.666738, -60.05) ccw construction
  line L47 (-31.934687, -58.05) -> (-33.934687, -58.05) construction
  ellipse E35 centre (-33.934687, -60.05) end of major axis (-33.934687, -58.05) minor radius 1.732051 (-33.934687, -58.05) -> (-35.666738, -60.05) ccw
  line L48 (-33.666738, -60.05) -> (-35.666738, -60.05) construction
  ellipse E36 centre (-30.578838, -2) end of major axis (-30.578838, -4) minor radius 1.732051 (-30.578838, -4) -> (-28.846788, -2) ccw
  line L49 (-30.578838, -4) -> (-34.04294, -4) construction
  ellipse E37 centre (-34.04294, -2) end of major axis (-34.04294, 0) minor radius 1.732051 (-35.774991, -2) -> (-34.04294, -4) ccw construction
  line L50 (-35.774991, -2) -> (-35.774991, 2) construction
  ellipse E38 centre (-34.04294, 2) end of major axis (-34.04294, 4) minor radius 1.732051 (-34.04294, 4) -> (-35.774991, 2) ccw construction
  line L51 (-34.04294, 4) -> (-30.578838, 4) construction
  ellipse E39 centre (-30.578838, 2) end of major axis (-30.578838, 0) minor radius 1.732051 (-28.846788, 2) -> (-30.578838, 4) ccw
  line L52 (-28.846788, 2) -> (-28.846788, -2)
  ellipse E40 centre (-32.310889, 0) end of major axis (-32.310889, 1.9) minor radius 1.645448 construction
  ellipse E41 centre (-30.470585, -60.05) end of major axis (-30.470585, -62.05) minor radius 1.732051 (-28.738534, -60.05) -> (-30.470585, -58.05) ccw
  line L53 (-28.738534, -60.05) -> (-28.738534, -64.05)
  ellipse E42 centre (-30.470585, -64.05) end of major axis (-30.470585, -66.05) minor radius 1.732051 (-30.470585, -66.05) -> (-28.738534, -64.05) ccw
  line L54 (-30.470585, -66.05) -> (-33.934687, -66.05) construction
  ellipse E43 centre (-33.934687, -64.05) end of major axis (-33.934687, -62.05) minor radius 1.732051 (-35.666738, -64.05) -> (-33.934687, -66.05) ccw construction
  line L55 (-35.666738, -64.05) -> (-35.666738, -60.05)
  ellipse E44 centre (-33.934687, -60.05) end of major axis (-33.934687, -58.05) minor radius 1.732051 (-33.934687, -58.05) -> (-35.666738, -60.05) ccw construction
  line L56 (-33.934687, -58.05) -> (-30.470585, -58.05) construction
  ellipse E45 centre (-32.202636, -62.05) end of major axis (-32.202636, -60.15) minor radius 1.645448 construction
  ellipse E46 centre (-5.464102, 0) end of major axis (-5.464102, 1.9) minor radius 1.645448 construction
  ellipse E47 centre (-172.082957, -31) end of major axis (-350.48419, -31) minor radius 103 (-2, 0.084764) -> (-4.29738, 4) ccw construction
  line L57 (-2, 0.084764) -> (-2, -2) construction
  ellipse E48 centre (-3.732051, -2) end of major axis (-3.732051, -4) minor radius 1.732051 (-3.732051, -4) -> (-2, -2) ccw construction
  line L58 (-3.732051, -4) -> (-7.196152, -4) construction
  ellipse E49 centre (-7.196152, -2) end of major axis (-7.196152, 0) minor radius 1.732051 (-8.928203, -2) -> (-7.196152, -4) ccw construction
  line L59 (-8.928203, -2) -> (-8.928203, 2) construction
  ellipse E50 centre (-7.196152, 2) end of major axis (-7.196152, 4) minor radius 1.732051 (-7.196152, 4) -> (-8.928203, 2) ccw construction
  line L60 (-7.196152, 4) -> (-4.29738, 4)
  ellipse E51 centre (-5.572355, -62.05) end of major axis (-5.572355, -60.15) minor radius 1.645448 construction
  ellipse E52 centre (-172.082957, -31) end of major axis (-350.48419, -31) minor radius 103 (-4.328695, -66.05) -> (-2.108253, -62.281517) ccw construction
  line L61 (-4.328695, -66.05) -> (-7.304406, -66.05)
  ellipse E53 centre (-7.304406, -64.05) end of major axis (-7.304406, -62.05) minor radius 1.732051 (-9.036456, -64.05) -> (-7.304406, -66.05) ccw construction
  line L62 (-9.036456, -64.05) -> (-9.036456, -60.05) construction
  ellipse E54 centre (-7.304406, -60.05) end of major axis (-7.304406, -58.05) minor radius 1.732051 (-7.304406, -58.05) -> (-9.036456, -60.05) ccw construction
  line L63 (-7.304406, -58.05) -> (-3.840304, -58.05)
  ellipse E55 centre (-3.840304, -60.05) end of major axis (-3.840304, -62.05) minor radius 1.732051 (-2.108253, -60.05) -> (-3.840304, -58.05) ccw construction
  line L64 (-2.108253, -60.05) -> (-2.108253, -62.281517) construction
  line L65 (-34.208003, -27.5) -> (-34.208003, 11.848348)
  line L66 (-34.208003, -73.848348) -> (-34.208003, -34.5)
  point P0 (-36.208003, -31)
  point P1 (-30.470585, -58.05)
  point P2 (-30.578838, -4)
  point P3 (-35.774991, -2)
  point P4 (-34.208003, -3.990897)
  point P5 (-34.208003, 3.990897)
  point P6 (-35.666738, -64.05)
  point P7 (-34.208003, -66.024942)
  point P8 (-34.208003, -58.075058)
  point P9 (-8.928203, 2)
  point P10 (-8.928203, -2)
  constraints: 52 other
extrude "Выдавливание13" add sketch "Эскиз13" along normal blind 16 and the other way blind 8 contours E39 L52 E36 L7 E8 L6 E7 L5 | E41 L53 E42 L38 E29 L37 E28 L36
extrude "Выдавливание14" cut sketch "Эскиз13" along normal blind 20 contours L10 E13 L65 E11 | L55 E35 L66 E33
extrude "Выдавливание15" add sketch "Эскиз13" against normal blind 20 contours L3 L23 E17 L20 E15 L60 L1 E1 L0 E0 | L61 E26 L30 E24 L63 L26 E20 L25 E19 L24
extrude "Выдавливание16" cut sketch "Эскиз12" against normal blind 4 contours A0 | A1 | A2 | A3
sketch "Эскиз14" plane through (0, 37, 0) normal (0, 1, 0) x (1, 0, 0)
  arc A0 (-93.050296, 48.648149) -> (-93.050296, -48.648149) centre (0, 0) ccw
  arc A1 (-93.050296, 48.648149) -> (-93.050296, -48.648149) centre (0, 0) ccw
  line L0 (-96.957897, 40.300945) -> (-125.520129, 38.609178)
  line L1 (-125.520129, 38.609178) -> (-122.280889, -45.476098)
  line L2 (-122.280889, -45.476098) -> (-97.199958, -39.713577)
  constraints: 6 end point, 2 point on circle
extrude "Выдавливание17" cut sketch "Эскиз14" against normal blind 36
